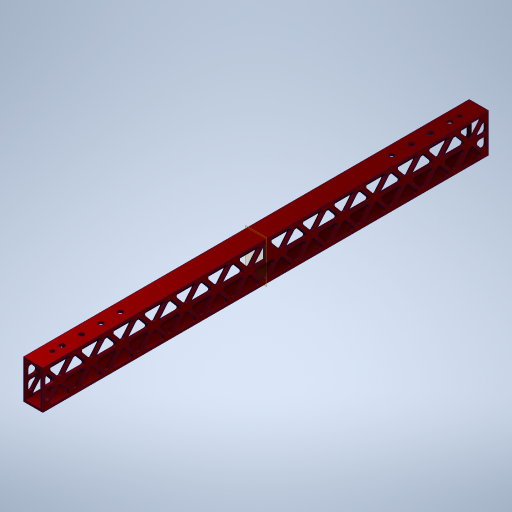
# Autodesk Inventor part: Drivetrain-Right-Left-Extrusion
Saved by Autodesk Inventor 2024.2 (Build 282272000, 272)
## iProperties
Created: 2024-01-04
Part Number: Drivetrain-Right-Left-Extrusion
Material: Aluminum 6061
Document SubType Name: Modeling
Designer: rohan
Density: 2.7 g/cm^3
Appearance: Aluminum - Flat
Author: rohan
Autodesk Inventor part; units mm, degrees
ref_plane "YZ Plane" through (0, 0, 0) normal (1, 0, 0) x (0, 1, 0)
ref_plane "XZ Plane" through (0, 0, 0) normal (0, 1, 0) x (-1, 0, 0)
ref_plane "XY Plane" through (0, 0, 0) normal (0, 0, 1) x (1, 0, 0)
sketch "Sketch1" plane through (0, 0, 0) normal (0, 0, 1) x (1, 0, 0)
  line L0 (-12.7, -25.4) -> (12.7, -25.4)
  line L1 (12.7, -25.4) -> (12.7, 25.4)
  line L2 (12.7, 25.4) -> (-12.7, 25.4)
  line L3 (-12.7, 25.4) -> (-12.7, -25.4)
  line L4 (-12.7, -25.4) -> (12.7, 25.4) construction
  line L5 (12.7, -25.4) -> (-12.7, 25.4) construction
  line L6 (-9.525, -22.225) -> (9.525, -22.225)
  line L7 (9.525, -22.225) -> (9.525, 22.225)
  line L8 (9.525, 22.225) -> (-9.525, 22.225)
  line L9 (-9.525, 22.225) -> (-9.525, -22.225)
  point P0 (0, 0)
  dimension "d0" = 25.4
  dimension "d1" = 50.8
  dimension "d2" = 3.175
  constraints: 20 end point, 4 parallel, 2 midpoint, 2 perpendicular, 1 horizontal, 3 other
  measures "d0" distance of L2.end L1.end
  measures "d1" distance of L1.end L0.end
  measures "d2" distance between parallel lines of L3 L9
extrude "Extrusion1" add sketch "Sketch1" along normal blind 584.2
sketch "Sketch2" plane through (-12.7, 25.4, 0) normal (0, 1, 0) x (1, 0, 0)
  circle A0 centre (12.7, -25.4) radius 2.5527
  circle A1 centre (12.7, -38.1) radius 3.2639
  line L0 (25.4, 0) -> (25.4, -584.2) projected
  circle A2 centre (12.7, -63.5) radius 3.2639
  circle A3 centre (12.7, -88.9) radius 3.2639
  circle A4 centre (12.7, -114.3) radius 3.2639
  point P0 (12.7, 0)
  dimension "d5" = 5.1054
  dimension "d6" = 25.4
  dimension "d7" = 6.5278
  dimension "d8" = 38.1
  dimension "d11" = 25.4
  constraints: 5 centre point, 1 vertical, 6 other
  measures "d5" diameter of A0
  measures "d6" distance of A0.centre point (12.7, 0)
  measures "d7" diameter of A1
  measures "d8" distance of A1.centre point (12.7, 0)
  measures "d11" distance of A1.centre A2.centre
extrude "Extrusion2" cut sketch "Sketch2" against normal blind 33.3375
ref_plane "Work Plane1" through (0, 0, 292.1) normal (0, 0, 1) x (1, 0, 0)
mirror "Mirror1" about plane through (0, 0, 292.1) normal (0, 0, 1) of "Extrusion2"
sketch "Sketch5" plane through (12.7, -25.4, 0) normal (1, 0, 0) x (0, 0, -1)
  line L0 (-584.2, 0) -> (-584.2, 50.8) projected
  line L1 (-584.2, 25.4) -> (0, 25.4)
  line L2 (-571.4463, 47.625) -> (-550.8435, 47.625)
  line L3 (-559.381, 30.6672) -> (-548.524, 42.2819)
  line L4 (0, 50.8) -> (-584.2, 50.8) projected
  line L5 (-564.1326, 30.7944) -> (-573.8785, 42.4091)
  arc A0 (-564.1326, 30.7944) -> (-559.381, 30.6672) centre (-561.7004, 32.8353) ccw
  arc A1 (-548.524, 42.2819) -> (-550.8435, 47.625) centre (-550.8435, 44.45) ccw
  arc A2 (-571.4463, 47.625) -> (-573.8785, 42.4091) centre (-571.4463, 44.45) ccw
  line L6 (-571.8917, 23.8125) -> (-577.85, 23.8125)
  line L7 (-569.4595, 18.5966) -> (-575.4178, 11.4958)
  line L8 (-581.025, 20.6375) -> (-581.025, 13.5367)
  line L9 (-571.8917, 26.9875) -> (-577.85, 26.9875)
  line L10 (-569.4595, 32.2034) -> (-575.4178, 39.3042)
  line L11 (-581.025, 30.1625) -> (-581.025, 37.2633)
  arc A3 (-575.4178, 39.3042) -> (-581.025, 37.2633) centre (-577.85, 37.2633) ccw
  arc A4 (-581.025, 30.1625) -> (-577.85, 26.9875) centre (-577.85, 30.1625) ccw
  arc A5 (-571.8917, 26.9875) -> (-569.4595, 32.2034) centre (-571.8917, 30.1625) ccw
  arc A6 (-577.85, 23.8125) -> (-581.025, 20.6375) centre (-577.85, 20.6375) ccw
  arc A7 (-569.4595, 18.5966) -> (-571.8917, 23.8125) centre (-571.8917, 20.6375) ccw
  arc A8 (-581.025, 13.5367) -> (-575.4178, 11.4958) centre (-577.85, 13.5367) ccw
  line L12 (-571.4463, 3.175) -> (-551.9485, 3.175)
  line L13 (-292.1, 50.8) -> (-292.1, 0)
  line L14 (0, 25.4) -> (-584.2, 25.4)
  line L15 (-542.6903, 6.0602) -> (-542.7392, 6.1185)
  line L16 (-564.1326, 20.0056) -> (-564.1356, 20.002)
  line L17 (-571.4463, 3.175) -> (-551.9605, 3.175)
  line L18 (-563.4572, 3.175) -> (-571.4463, 3.175)
  line L19 (-564.1356, 20.002) -> (-573.8785, 8.3909)
  line L20 (-559.2712, 20.002) -> (-549.5283, 8.3909)
  line L21 (-564.1356, 20.002) -> (-559.1614, 20.002) construction
  line L22 (-559.2712, 20.002) -> (-554.4261, 20.002) construction
  arc A9 (-573.8785, 8.3909) -> (-571.4463, 3.175) centre (-571.4463, 6.35) ccw
  arc A10 (-551.9605, 3.175) -> (-549.5283, 8.3909) centre (-551.9605, 6.35) ccw
  arc A11 (-559.2712, 20.002) -> (-564.1356, 20.002) centre (-561.7034, 17.9612) ccw
  line L23 (0, 0) -> (-584.2, 0) projected
  line L24 (-558.9257, 19.5902) -> (-549.5283, 8.3909)
  line L25 (-553.9473, 18.5966) -> (-547.0961, 10.4317)
  line L26 (-543.6299, 23.8125) -> (-551.5151, 23.8125)
  line L27 (-553.9473, 18.5966) -> (-544.208, 6.9898)
  line L28 (-543.6299, 23.8125) -> (-531.1495, 23.8125)
  line L29 (-551.5151, 23.8125) -> (-532.0365, 23.8125)
  line L30 (-529.6043, 18.5966) -> (-539.3436, 6.9898)
  arc A12 (-544.208, 6.9898) -> (-539.3436, 6.9898) centre (-541.7758, 9.0307) ccw
  arc A13 (-551.5151, 23.8125) -> (-553.9473, 18.5966) centre (-551.5151, 20.6375) ccw
  arc A14 (-529.6043, 18.5966) -> (-532.0365, 23.8125) centre (-532.0365, 20.6375) ccw
  line L31 (-557.5436, 23.8125) -> (-557.5862, 23.8125)
  line L32 (-558.2741, 23.8125) -> (-558.3239, 23.8125)
  line L33 (-553.9473, 32.2034) -> (-544.208, 43.8102)
  line L34 (-551.5151, 26.9875) -> (-532.0365, 26.9875)
  line L35 (-529.6043, 32.2034) -> (-539.3436, 43.8102)
  arc A15 (-539.3436, 43.8102) -> (-544.208, 43.8102) centre (-541.7758, 41.7693) ccw
  arc A16 (-553.9473, 32.2034) -> (-551.5151, 26.9875) centre (-551.5151, 30.1625) ccw
  arc A17 (-532.0365, 26.9875) -> (-529.6043, 32.2034) centre (-532.0365, 30.1625) ccw
  line L36 (-12.7537, 47.625) -> (-33.3565, 47.625)
  line L37 (-24.819, 30.6672) -> (-35.676, 42.2819)
  line L38 (-20.0674, 30.7944) -> (-10.3215, 42.4091)
  arc A18 (-24.819, 30.6672) -> (-20.0674, 30.7944) centre (-22.4996, 32.8353) ccw
  arc A19 (-33.3565, 47.625) -> (-35.676, 42.2819) centre (-33.3565, 44.45) ccw
  arc A20 (-10.3215, 42.4091) -> (-12.7537, 47.625) centre (-12.7537, 44.45) ccw
  line L39 (-12.3083, 23.8125) -> (-6.35, 23.8125)
  line L40 (-14.7405, 18.5966) -> (-8.7822, 11.4958)
  line L41 (-3.175, 20.6375) -> (-3.175, 13.5367)
  line L42 (-12.3083, 26.9875) -> (-6.35, 26.9875)
  line L43 (-3.175, 30.1625) -> (-3.175, 37.2633)
  line L44 (-14.7405, 32.2034) -> (-8.7822, 39.3042)
  arc A21 (-3.175, 37.2633) -> (-8.7822, 39.3042) centre (-6.35, 37.2633) ccw
  arc A22 (-6.35, 26.9875) -> (-3.175, 30.1625) centre (-6.35, 30.1625) ccw
  arc A23 (-14.7405, 32.2034) -> (-12.3083, 26.9875) centre (-12.3083, 30.1625) ccw
  arc A24 (-3.175, 20.6375) -> (-6.35, 23.8125) centre (-6.35, 20.6375) ccw
  arc A25 (-12.3083, 23.8125) -> (-14.7405, 18.5966) centre (-12.3083, 20.6375) ccw
  arc A26 (-8.7822, 11.4958) -> (-3.175, 13.5367) centre (-6.35, 13.5367) ccw
  line L45 (-12.7537, 3.175) -> (-32.2515, 3.175)
  line L46 (-20.0674, 20.0056) -> (-20.0644, 20.002)
  line L47 (-20.7428, 3.175) -> (-12.7537, 3.175)
  line L48 (-20.0644, 20.002) -> (-10.3215, 8.3909)
  line L49 (-24.9288, 20.002) -> (-34.6717, 8.3909)
  line L50 (-20.0644, 20.002) -> (-25.0386, 20.002) construction
  line L51 (-24.9288, 20.002) -> (-29.7739, 20.002) construction
  arc A27 (-12.7537, 3.175) -> (-10.3215, 8.3909) centre (-12.7537, 6.35) ccw
  arc A28 (-34.6717, 8.3909) -> (-32.2395, 3.175) centre (-32.2395, 6.35) ccw
  arc A29 (-20.0644, 20.002) -> (-24.9288, 20.002) centre (-22.4966, 17.9612) ccw
  line L52 (-26.6564, 23.8125) -> (-26.6138, 23.8125)
  line L53 (-25.9259, 23.8125) -> (-25.8761, 23.8125)
  line L54 (41.402, 25.4) -> (-542.798, 25.4)
  arc A30 (-522.7306, 30.7944) -> (-517.979, 30.6672) centre (-520.2984, 32.8353) ccw
  line L55 (-517.979, 30.6672) -> (-507.122, 42.2819)
  line L56 (-522.7306, 30.7944) -> (-532.4765, 42.4091)
  arc A31 (-507.122, 42.2819) -> (-509.4415, 47.625) centre (-509.4415, 44.45) ccw
  line L57 (-530.0443, 47.625) -> (-509.4415, 47.625)
  line L58 (-517.8692, 20.002) -> (-513.0241, 20.002) construction
  line L59 (-522.7336, 20.002) -> (-517.7594, 20.002) construction
  line L60 (-517.8692, 20.002) -> (-508.1263, 8.3909)
  arc A32 (-510.5585, 3.175) -> (-508.1263, 8.3909) centre (-510.5585, 6.35) ccw
  line L61 (-530.0443, 3.175) -> (-510.5465, 3.175)
  line L62 (-530.0443, 3.175) -> (-510.5585, 3.175)
  line L63 (-522.7336, 20.002) -> (-532.4765, 8.3909)
  line L64 (-522.0552, 3.175) -> (-530.0443, 3.175)
  arc A33 (-517.8692, 20.002) -> (-522.7336, 20.002) centre (-520.3014, 17.9612) ccw
  line L65 (-522.7306, 20.0056) -> (-522.7336, 20.002)
  line L66 (-501.2883, 6.0602) -> (-501.3372, 6.1185)
  line L67 (-517.5237, 19.5902) -> (-508.1263, 8.3909)
  line L68 (-512.5453, 18.5966) -> (-505.6941, 10.4317)
  line L69 (-502.2279, 23.8125) -> (-510.1131, 23.8125)
  line L70 (-512.5453, 18.5966) -> (-502.806, 6.9898)
  arc A34 (-488.2023, 18.5966) -> (-490.6345, 23.8125) centre (-490.6345, 20.6375) ccw
  arc A35 (-502.806, 6.9898) -> (-497.9416, 6.9898) centre (-500.3738, 9.0307) ccw
  line L71 (-488.2023, 18.5966) -> (-497.9416, 6.9898)
  line L72 (-502.2279, 23.8125) -> (-489.7475, 23.8125)
  arc A36 (-510.1131, 23.8125) -> (-512.5453, 18.5966) centre (-510.1131, 20.6375) ccw
  line L73 (-510.1131, 23.8125) -> (-490.6345, 23.8125)
  line L74 (-516.1416, 23.8125) -> (-516.1842, 23.8125)
  line L75 (-516.8721, 23.8125) -> (-516.9219, 23.8125)
  arc A37 (-490.6345, 26.9875) -> (-488.2023, 32.2034) centre (-490.6345, 30.1625) ccw
  line L76 (-510.1131, 26.9875) -> (-490.6345, 26.9875)
  arc A38 (-512.5453, 32.2034) -> (-510.1131, 26.9875) centre (-510.1131, 30.1625) ccw
  line L77 (-488.2023, 32.2034) -> (-497.9416, 43.8102)
  line L78 (-512.5453, 32.2034) -> (-502.806, 43.8102)
  arc A39 (-497.9416, 43.8102) -> (-502.806, 43.8102) centre (-500.3738, 41.7693) ccw
  arc A40 (-532.4765, 8.3909) -> (-530.0443, 3.175) centre (-530.0443, 6.35) ccw
  arc A41 (-530.0443, 47.625) -> (-532.4765, 42.4091) centre (-530.0443, 44.45) ccw
  line L79 (82.804, 25.4) -> (-501.396, 25.4)
  arc A42 (-481.3286, 30.7944) -> (-476.577, 30.6672) centre (-478.8964, 32.8353) ccw
  line L80 (-476.577, 30.6672) -> (-465.72, 42.2819)
  line L81 (-481.3286, 30.7944) -> (-491.0745, 42.4091)
  arc A43 (-465.72, 42.2819) -> (-468.0395, 47.625) centre (-468.0395, 44.45) ccw
  line L82 (-488.6423, 47.625) -> (-468.0395, 47.625)
  line L83 (-476.4672, 20.002) -> (-471.6221, 20.002) construction
  line L84 (-481.3316, 20.002) -> (-476.3574, 20.002) construction
  line L85 (-476.4672, 20.002) -> (-466.7243, 8.3909)
  arc A44 (-469.1565, 3.175) -> (-466.7243, 8.3909) centre (-469.1565, 6.35) ccw
  line L86 (-488.6423, 3.175) -> (-469.1445, 3.175)
  line L87 (-488.6423, 3.175) -> (-469.1565, 3.175)
  line L88 (-481.3316, 20.002) -> (-491.0745, 8.3909)
  line L89 (-480.6532, 3.175) -> (-488.6423, 3.175)
  arc A45 (-476.4672, 20.002) -> (-481.3316, 20.002) centre (-478.8994, 17.9612) ccw
  line L90 (-481.3286, 20.0056) -> (-481.3316, 20.002)
  line L91 (-459.8863, 6.0602) -> (-459.9352, 6.1185)
  line L92 (-476.1217, 19.5902) -> (-466.7243, 8.3909)
  line L93 (-471.1433, 18.5966) -> (-464.2921, 10.4317)
  line L94 (-460.8259, 23.8125) -> (-468.7111, 23.8125)
  line L95 (-471.1433, 18.5966) -> (-461.404, 6.9898)
  arc A46 (-446.8003, 18.5966) -> (-449.2325, 23.8125) centre (-449.2325, 20.6375) ccw
  arc A47 (-461.404, 6.9898) -> (-456.5396, 6.9898) centre (-458.9718, 9.0307) ccw
  line L96 (-446.8003, 18.5966) -> (-456.5396, 6.9898)
  line L97 (-460.8259, 23.8125) -> (-448.3455, 23.8125)
  arc A48 (-468.7111, 23.8125) -> (-471.1433, 18.5966) centre (-468.7111, 20.6375) ccw
  line L98 (-468.7111, 23.8125) -> (-449.2325, 23.8125)
  line L99 (-474.7396, 23.8125) -> (-474.7822, 23.8125)
  line L100 (-475.4701, 23.8125) -> (-475.5199, 23.8125)
  arc A49 (-449.2325, 26.9875) -> (-446.8003, 32.2034) centre (-449.2325, 30.1625) ccw
  line L101 (-468.7111, 26.9875) -> (-449.2325, 26.9875)
  arc A50 (-471.1433, 32.2034) -> (-468.7111, 26.9875) centre (-468.7111, 30.1625) ccw
  line L102 (-446.8003, 32.2034) -> (-456.5396, 43.8102)
  line L103 (-471.1433, 32.2034) -> (-461.404, 43.8102)
  arc A51 (-456.5396, 43.8102) -> (-461.404, 43.8102) centre (-458.9718, 41.7693) ccw
  arc A52 (-491.0745, 8.3909) -> (-488.6423, 3.175) centre (-488.6423, 6.35) ccw
  arc A53 (-488.6423, 47.625) -> (-491.0745, 42.4091) centre (-488.6423, 44.45) ccw
  line L104 (124.206, 25.4) -> (-459.994, 25.4)
  arc A54 (-439.9266, 30.7944) -> (-435.175, 30.6672) centre (-437.4944, 32.8353) ccw
  line L105 (-435.175, 30.6672) -> (-424.318, 42.2819)
  line L106 (-439.9266, 30.7944) -> (-449.6725, 42.4091)
  arc A55 (-424.318, 42.2819) -> (-426.6375, 47.625) centre (-426.6375, 44.45) ccw
  line L107 (-447.2403, 47.625) -> (-426.6375, 47.625)
  line L108 (-435.0652, 20.002) -> (-430.2201, 20.002) construction
  line L109 (-439.9296, 20.002) -> (-434.9554, 20.002) construction
  line L110 (-435.0652, 20.002) -> (-425.3223, 8.3909)
  arc A56 (-427.7545, 3.175) -> (-425.3223, 8.3909) centre (-427.7545, 6.35) ccw
  line L111 (-447.2403, 3.175) -> (-427.7425, 3.175)
  line L112 (-447.2403, 3.175) -> (-427.7545, 3.175)
  line L113 (-439.9296, 20.002) -> (-449.6725, 8.3909)
  line L114 (-439.2512, 3.175) -> (-447.2403, 3.175)
  arc A57 (-435.0652, 20.002) -> (-439.9296, 20.002) centre (-437.4974, 17.9612) ccw
  line L115 (-439.9266, 20.0056) -> (-439.9296, 20.002)
  line L116 (-418.4843, 6.0602) -> (-418.5332, 6.1185)
  line L117 (-434.7197, 19.5902) -> (-425.3223, 8.3909)
  line L118 (-429.7413, 18.5966) -> (-422.8901, 10.4317)
  line L119 (-419.4239, 23.8125) -> (-427.3091, 23.8125)
  line L120 (-429.7413, 18.5966) -> (-420.002, 6.9898)
  arc A58 (-405.3983, 18.5966) -> (-407.8305, 23.8125) centre (-407.8305, 20.6375) ccw
  arc A59 (-420.002, 6.9898) -> (-415.1376, 6.9898) centre (-417.5698, 9.0307) ccw
  line L121 (-405.3983, 18.5966) -> (-415.1376, 6.9898)
  line L122 (-419.4239, 23.8125) -> (-406.9435, 23.8125)
  arc A60 (-427.3091, 23.8125) -> (-429.7413, 18.5966) centre (-427.3091, 20.6375) ccw
  line L123 (-427.3091, 23.8125) -> (-407.8305, 23.8125)
  line L124 (-433.3376, 23.8125) -> (-433.3802, 23.8125)
  line L125 (-434.0681, 23.8125) -> (-434.1179, 23.8125)
  arc A61 (-407.8305, 26.9875) -> (-405.3983, 32.2034) centre (-407.8305, 30.1625) ccw
  line L126 (-427.3091, 26.9875) -> (-407.8305, 26.9875)
  arc A62 (-429.7413, 32.2034) -> (-427.3091, 26.9875) centre (-427.3091, 30.1625) ccw
  line L127 (-405.3983, 32.2034) -> (-415.1376, 43.8102)
  line L128 (-429.7413, 32.2034) -> (-420.002, 43.8102)
  arc A63 (-415.1376, 43.8102) -> (-420.002, 43.8102) centre (-417.5698, 41.7693) ccw
  arc A64 (-449.6725, 8.3909) -> (-447.2403, 3.175) centre (-447.2403, 6.35) ccw
  arc A65 (-447.2403, 47.625) -> (-449.6725, 42.4091) centre (-447.2403, 44.45) ccw
  line L129 (165.608, 25.4) -> (-418.592, 25.4)
  arc A66 (-398.5246, 30.7944) -> (-393.773, 30.6672) centre (-396.0924, 32.8353) ccw
  line L130 (-393.773, 30.6672) -> (-382.916, 42.2819)
  line L131 (-398.5246, 30.7944) -> (-408.2705, 42.4091)
  arc A67 (-382.916, 42.2819) -> (-385.2355, 47.625) centre (-385.2355, 44.45) ccw
  line L132 (-405.8383, 47.625) -> (-385.2355, 47.625)
  line L133 (-393.6632, 20.002) -> (-388.8181, 20.002) construction
  line L134 (-398.5276, 20.002) -> (-393.5534, 20.002) construction
  line L135 (-393.6632, 20.002) -> (-383.9203, 8.3909)
  arc A68 (-386.3525, 3.175) -> (-383.9203, 8.3909) centre (-386.3525, 6.35) ccw
  line L136 (-405.8383, 3.175) -> (-386.3405, 3.175)
  line L137 (-405.8383, 3.175) -> (-386.3525, 3.175)
  line L138 (-398.5276, 20.002) -> (-408.2705, 8.3909)
  line L139 (-397.8492, 3.175) -> (-405.8383, 3.175)
  arc A69 (-393.6632, 20.002) -> (-398.5276, 20.002) centre (-396.0954, 17.9612) ccw
  line L140 (-398.5246, 20.0056) -> (-398.5276, 20.002)
  line L141 (-377.0823, 6.0602) -> (-377.1312, 6.1185)
  line L142 (-393.3177, 19.5902) -> (-383.9203, 8.3909)
  line L143 (-388.3393, 18.5966) -> (-381.4881, 10.4317)
  line L144 (-378.0219, 23.8125) -> (-385.9071, 23.8125)
  line L145 (-388.3393, 18.5966) -> (-378.6, 6.9898)
  arc A70 (-363.9963, 18.5966) -> (-366.4285, 23.8125) centre (-366.4285, 20.6375) ccw
  arc A71 (-378.6, 6.9898) -> (-373.7356, 6.9898) centre (-376.1678, 9.0307) ccw
  line L146 (-363.9963, 18.5966) -> (-373.7356, 6.9898)
  line L147 (-378.0219, 23.8125) -> (-365.5415, 23.8125)
  arc A72 (-385.9071, 23.8125) -> (-388.3393, 18.5966) centre (-385.9071, 20.6375) ccw
  line L148 (-385.9071, 23.8125) -> (-366.4285, 23.8125)
  line L149 (-391.9356, 23.8125) -> (-391.9782, 23.8125)
  line L150 (-392.6661, 23.8125) -> (-392.7159, 23.8125)
  arc A73 (-366.4285, 26.9875) -> (-363.9963, 32.2034) centre (-366.4285, 30.1625) ccw
  line L151 (-385.9071, 26.9875) -> (-366.4285, 26.9875)
  arc A74 (-388.3393, 32.2034) -> (-385.9071, 26.9875) centre (-385.9071, 30.1625) ccw
  line L152 (-363.9963, 32.2034) -> (-373.7356, 43.8102)
  line L153 (-388.3393, 32.2034) -> (-378.6, 43.8102)
  arc A75 (-373.7356, 43.8102) -> (-378.6, 43.8102) centre (-376.1678, 41.7693) ccw
  arc A76 (-408.2705, 8.3909) -> (-405.8383, 3.175) centre (-405.8383, 6.35) ccw
  arc A77 (-405.8383, 47.625) -> (-408.2705, 42.4091) centre (-405.8383, 44.45) ccw
  line L154 (207.01, 25.4) -> (-377.19, 25.4)
  arc A78 (-357.1226, 30.7944) -> (-352.371, 30.6672) centre (-354.6904, 32.8353) ccw
  line L155 (-352.371, 30.6672) -> (-341.514, 42.2819)
  line L156 (-357.1226, 30.7944) -> (-366.8685, 42.4091)
  arc A79 (-341.514, 42.2819) -> (-343.8335, 47.625) centre (-343.8335, 44.45) ccw
  line L157 (-364.4363, 47.625) -> (-343.8335, 47.625)
  line L158 (-352.2612, 20.002) -> (-347.4161, 20.002) construction
  line L159 (-357.1256, 20.002) -> (-352.1514, 20.002) construction
  line L160 (-352.2612, 20.002) -> (-342.5183, 8.3909)
  arc A80 (-344.9505, 3.175) -> (-342.5183, 8.3909) centre (-344.9505, 6.35) ccw
  line L161 (-364.4363, 3.175) -> (-344.9385, 3.175)
  line L162 (-364.4363, 3.175) -> (-344.9505, 3.175)
  line L163 (-357.1256, 20.002) -> (-366.8685, 8.3909)
  line L164 (-356.4472, 3.175) -> (-364.4363, 3.175)
  arc A81 (-352.2612, 20.002) -> (-357.1256, 20.002) centre (-354.6934, 17.9612) ccw
  line L165 (-357.1226, 20.0056) -> (-357.1256, 20.002)
  line L166 (-335.6803, 6.0602) -> (-335.7292, 6.1185)
  line L167 (-351.9157, 19.5902) -> (-342.5183, 8.3909)
  line L168 (-346.9373, 18.5966) -> (-340.0861, 10.4317)
  line L169 (-336.6199, 23.8125) -> (-344.5051, 23.8125)
  line L170 (-346.9373, 18.5966) -> (-337.198, 6.9898)
  arc A82 (-322.5943, 18.5966) -> (-325.0265, 23.8125) centre (-325.0265, 20.6375) ccw
  arc A83 (-337.198, 6.9898) -> (-332.3336, 6.9898) centre (-334.7658, 9.0307) ccw
  line L171 (-322.5943, 18.5966) -> (-332.3336, 6.9898)
  line L172 (-336.6199, 23.8125) -> (-324.1395, 23.8125)
  arc A84 (-344.5051, 23.8125) -> (-346.9373, 18.5966) centre (-344.5051, 20.6375) ccw
  line L173 (-344.5051, 23.8125) -> (-325.0265, 23.8125)
  line L174 (-350.5336, 23.8125) -> (-350.5762, 23.8125)
  line L175 (-351.2641, 23.8125) -> (-351.3139, 23.8125)
  arc A85 (-325.0265, 26.9875) -> (-322.5943, 32.2034) centre (-325.0265, 30.1625) ccw
  line L176 (-344.5051, 26.9875) -> (-325.0265, 26.9875)
  arc A86 (-346.9373, 32.2034) -> (-344.5051, 26.9875) centre (-344.5051, 30.1625) ccw
  line L177 (-322.5943, 32.2034) -> (-332.3336, 43.8102)
  line L178 (-346.9373, 32.2034) -> (-337.198, 43.8102)
  arc A87 (-332.3336, 43.8102) -> (-337.198, 43.8102) centre (-334.7658, 41.7693) ccw
  arc A88 (-366.8685, 8.3909) -> (-364.4363, 3.175) centre (-364.4363, 6.35) ccw
  arc A89 (-364.4363, 47.625) -> (-366.8685, 42.4091) centre (-364.4363, 44.45) ccw
  line L179 (248.412, 25.4) -> (-335.788, 25.4)
  arc A90 (-315.7206, 30.7944) -> (-310.969, 30.6672) centre (-313.2884, 32.8353) ccw
  line L180 (-310.969, 30.6672) -> (-300.112, 42.2819)
  line L181 (-315.7206, 30.7944) -> (-325.4665, 42.4091)
  arc A91 (-300.112, 42.2819) -> (-302.4315, 47.625) centre (-302.4315, 44.45) ccw
  line L182 (-323.0343, 47.625) -> (-302.4315, 47.625)
  line L183 (-310.8592, 20.002) -> (-306.0141, 20.002) construction
  line L184 (-315.7236, 20.002) -> (-310.7494, 20.002) construction
  line L185 (-310.8592, 20.002) -> (-301.1163, 8.3909)
  arc A92 (-303.5485, 3.175) -> (-301.1163, 8.3909) centre (-303.5485, 6.35) ccw
  line L186 (-323.0343, 3.175) -> (-303.5365, 3.175)
  line L187 (-323.0343, 3.175) -> (-303.5485, 3.175)
  line L188 (-315.7236, 20.002) -> (-325.4665, 8.3909)
  line L189 (-315.0452, 3.175) -> (-323.0343, 3.175)
  arc A93 (-310.8592, 20.002) -> (-315.7236, 20.002) centre (-313.2914, 17.9612) ccw
  line L190 (-315.7206, 20.0056) -> (-315.7236, 20.002)
  line L191 (-294.2783, 6.0602) -> (-294.3272, 6.1185)
  line L192 (-310.5137, 19.5902) -> (-301.1163, 8.3909)
  line L193 (-305.5353, 18.5966) -> (-298.6841, 10.4317)
  line L194 (-295.2179, 23.8125) -> (-303.1031, 23.8125)
  line L195 (-305.5353, 18.5966) -> (-295.796, 6.9898)
  arc A94 (-281.1923, 18.5966) -> (-283.6245, 23.8125) centre (-283.6245, 20.6375) ccw
  arc A95 (-295.796, 6.9898) -> (-290.9316, 6.9898) centre (-293.3638, 9.0307) ccw
  line L196 (-281.1923, 18.5966) -> (-290.9316, 6.9898)
  line L197 (-295.2179, 23.8125) -> (-282.7375, 23.8125)
  arc A96 (-303.1031, 23.8125) -> (-305.5353, 18.5966) centre (-303.1031, 20.6375) ccw
  line L198 (-303.1031, 23.8125) -> (-283.6245, 23.8125)
  line L199 (-309.1316, 23.8125) -> (-309.1742, 23.8125)
  line L200 (-309.8621, 23.8125) -> (-309.9119, 23.8125)
  arc A97 (-283.6245, 26.9875) -> (-281.1923, 32.2034) centre (-283.6245, 30.1625) ccw
  line L201 (-303.1031, 26.9875) -> (-283.6245, 26.9875)
  arc A98 (-305.5353, 32.2034) -> (-303.1031, 26.9875) centre (-303.1031, 30.1625) ccw
  line L202 (-281.1923, 32.2034) -> (-290.9316, 43.8102)
  line L203 (-305.5353, 32.2034) -> (-295.796, 43.8102)
  arc A99 (-290.9316, 43.8102) -> (-295.796, 43.8102) centre (-293.3638, 41.7693) ccw
  arc A100 (-325.4665, 8.3909) -> (-323.0343, 3.175) centre (-323.0343, 6.35) ccw
  arc A101 (-323.0343, 47.625) -> (-325.4665, 42.4091) centre (-323.0343, 44.45) ccw
  line L204 (289.814, 25.4) -> (-294.386, 25.4)
  arc A102 (-274.3186, 30.7944) -> (-269.567, 30.6672) centre (-271.8864, 32.8353) ccw
  line L205 (-269.567, 30.6672) -> (-258.71, 42.2819)
  line L206 (-274.3186, 30.7944) -> (-284.0645, 42.4091)
  arc A103 (-258.71, 42.2819) -> (-261.0295, 47.625) centre (-261.0295, 44.45) ccw
  line L207 (-281.6323, 47.625) -> (-261.0295, 47.625)
  line L208 (-269.4572, 20.002) -> (-264.6121, 20.002) construction
  line L209 (-274.3216, 20.002) -> (-269.3474, 20.002) construction
  line L210 (-269.4572, 20.002) -> (-259.7143, 8.3909)
  arc A104 (-262.1465, 3.175) -> (-259.7143, 8.3909) centre (-262.1465, 6.35) ccw
  line L211 (-281.6323, 3.175) -> (-262.1345, 3.175)
  line L212 (-281.6323, 3.175) -> (-262.1465, 3.175)
  line L213 (-274.3216, 20.002) -> (-284.0645, 8.3909)
  line L214 (-273.6432, 3.175) -> (-281.6323, 3.175)
  arc A105 (-269.4572, 20.002) -> (-274.3216, 20.002) centre (-271.8894, 17.9612) ccw
  line L215 (-274.3186, 20.0056) -> (-274.3216, 20.002)
  line L216 (-252.8763, 6.0602) -> (-252.9252, 6.1185)
  line L217 (-269.1117, 19.5902) -> (-259.7143, 8.3909)
  line L218 (-264.1333, 18.5966) -> (-257.2821, 10.4317)
  line L219 (-253.8159, 23.8125) -> (-261.7011, 23.8125)
  line L220 (-264.1333, 18.5966) -> (-254.394, 6.9898)
  arc A106 (-239.7903, 18.5966) -> (-242.2225, 23.8125) centre (-242.2225, 20.6375) ccw
  arc A107 (-254.394, 6.9898) -> (-249.5296, 6.9898) centre (-251.9618, 9.0307) ccw
  line L221 (-239.7903, 18.5966) -> (-249.5296, 6.9898)
  line L222 (-253.8159, 23.8125) -> (-241.3355, 23.8125)
  arc A108 (-261.7011, 23.8125) -> (-264.1333, 18.5966) centre (-261.7011, 20.6375) ccw
  line L223 (-261.7011, 23.8125) -> (-242.2225, 23.8125)
  line L224 (-267.7296, 23.8125) -> (-267.7722, 23.8125)
  line L225 (-268.4601, 23.8125) -> (-268.5099, 23.8125)
  arc A109 (-242.2225, 26.9875) -> (-239.7903, 32.2034) centre (-242.2225, 30.1625) ccw
  line L226 (-261.7011, 26.9875) -> (-242.2225, 26.9875)
  arc A110 (-264.1333, 32.2034) -> (-261.7011, 26.9875) centre (-261.7011, 30.1625) ccw
  line L227 (-239.7903, 32.2034) -> (-249.5296, 43.8102)
  line L228 (-264.1333, 32.2034) -> (-254.394, 43.8102)
  arc A111 (-249.5296, 43.8102) -> (-254.394, 43.8102) centre (-251.9618, 41.7693) ccw
  arc A112 (-284.0645, 8.3909) -> (-281.6323, 3.175) centre (-281.6323, 6.35) ccw
  arc A113 (-281.6323, 47.625) -> (-284.0645, 42.4091) centre (-281.6323, 44.45) ccw
  line L229 (331.216, 25.4) -> (-252.984, 25.4)
  arc A114 (-232.9166, 30.7944) -> (-228.165, 30.6672) centre (-230.4844, 32.8353) ccw
  line L230 (-228.165, 30.6672) -> (-217.308, 42.2819)
  line L231 (-232.9166, 30.7944) -> (-242.6625, 42.4091)
  arc A115 (-217.308, 42.2819) -> (-219.6275, 47.625) centre (-219.6275, 44.45) ccw
  line L232 (-240.2303, 47.625) -> (-219.6275, 47.625)
  line L233 (-228.0552, 20.002) -> (-223.2101, 20.002) construction
  line L234 (-232.9196, 20.002) -> (-227.9454, 20.002) construction
  line L235 (-228.0552, 20.002) -> (-218.3123, 8.3909)
  arc A116 (-220.7445, 3.175) -> (-218.3123, 8.3909) centre (-220.7445, 6.35) ccw
  line L236 (-240.2303, 3.175) -> (-220.7325, 3.175)
  line L237 (-240.2303, 3.175) -> (-220.7445, 3.175)
  line L238 (-232.9196, 20.002) -> (-242.6625, 8.3909)
  line L239 (-232.2412, 3.175) -> (-240.2303, 3.175)
  arc A117 (-228.0552, 20.002) -> (-232.9196, 20.002) centre (-230.4874, 17.9612) ccw
  line L240 (-232.9166, 20.0056) -> (-232.9196, 20.002)
  line L241 (-211.4743, 6.0602) -> (-211.5232, 6.1185)
  line L242 (-227.7097, 19.5902) -> (-218.3123, 8.3909)
  line L243 (-222.7313, 18.5966) -> (-215.8801, 10.4317)
  line L244 (-212.4139, 23.8125) -> (-220.2991, 23.8125)
  line L245 (-222.7313, 18.5966) -> (-212.992, 6.9898)
  arc A118 (-198.3883, 18.5966) -> (-200.8205, 23.8125) centre (-200.8205, 20.6375) ccw
  arc A119 (-212.992, 6.9898) -> (-208.1276, 6.9898) centre (-210.5598, 9.0307) ccw
  line L246 (-198.3883, 18.5966) -> (-208.1276, 6.9898)
  line L247 (-212.4139, 23.8125) -> (-199.9335, 23.8125)
  arc A120 (-220.2991, 23.8125) -> (-222.7313, 18.5966) centre (-220.2991, 20.6375) ccw
  line L248 (-220.2991, 23.8125) -> (-200.8205, 23.8125)
  line L249 (-226.3276, 23.8125) -> (-226.3702, 23.8125)
  line L250 (-227.0581, 23.8125) -> (-227.1079, 23.8125)
  arc A121 (-200.8205, 26.9875) -> (-198.3883, 32.2034) centre (-200.8205, 30.1625) ccw
  line L251 (-220.2991, 26.9875) -> (-200.8205, 26.9875)
  arc A122 (-222.7313, 32.2034) -> (-220.2991, 26.9875) centre (-220.2991, 30.1625) ccw
  line L252 (-198.3883, 32.2034) -> (-208.1276, 43.8102)
  line L253 (-222.7313, 32.2034) -> (-212.992, 43.8102)
  arc A123 (-208.1276, 43.8102) -> (-212.992, 43.8102) centre (-210.5598, 41.7693) ccw
  arc A124 (-242.6625, 8.3909) -> (-240.2303, 3.175) centre (-240.2303, 6.35) ccw
  arc A125 (-240.2303, 47.625) -> (-242.6625, 42.4091) centre (-240.2303, 44.45) ccw
  line L254 (372.618, 25.4) -> (-211.582, 25.4)
  arc A126 (-191.5146, 30.7944) -> (-186.763, 30.6672) centre (-189.0824, 32.8353) ccw
  line L255 (-186.763, 30.6672) -> (-175.906, 42.2819)
  line L256 (-191.5146, 30.7944) -> (-201.2605, 42.4091)
  arc A127 (-175.906, 42.2819) -> (-178.2255, 47.625) centre (-178.2255, 44.45) ccw
  line L257 (-198.8283, 47.625) -> (-178.2255, 47.625)
  line L258 (-186.6532, 20.002) -> (-181.8081, 20.002) construction
  line L259 (-191.5176, 20.002) -> (-186.5434, 20.002) construction
  line L260 (-186.6532, 20.002) -> (-176.9103, 8.3909)
  arc A128 (-179.3425, 3.175) -> (-176.9103, 8.3909) centre (-179.3425, 6.35) ccw
  line L261 (-198.8283, 3.175) -> (-179.3305, 3.175)
  line L262 (-198.8283, 3.175) -> (-179.3425, 3.175)
  line L263 (-191.5176, 20.002) -> (-201.2605, 8.3909)
  line L264 (-190.8392, 3.175) -> (-198.8283, 3.175)
  arc A129 (-186.6532, 20.002) -> (-191.5176, 20.002) centre (-189.0854, 17.9612) ccw
  line L265 (-191.5146, 20.0056) -> (-191.5176, 20.002)
  line L266 (-170.0723, 6.0602) -> (-170.1212, 6.1185)
  line L267 (-186.3077, 19.5902) -> (-176.9103, 8.3909)
  line L268 (-181.3293, 18.5966) -> (-174.4781, 10.4317)
  line L269 (-171.0119, 23.8125) -> (-178.8971, 23.8125)
  line L270 (-181.3293, 18.5966) -> (-171.59, 6.9898)
  arc A130 (-156.9863, 18.5966) -> (-159.4185, 23.8125) centre (-159.4185, 20.6375) ccw
  arc A131 (-171.59, 6.9898) -> (-166.7256, 6.9898) centre (-169.1578, 9.0307) ccw
  line L271 (-156.9863, 18.5966) -> (-166.7256, 6.9898)
  line L272 (-171.0119, 23.8125) -> (-158.5315, 23.8125)
  arc A132 (-178.8971, 23.8125) -> (-181.3293, 18.5966) centre (-178.8971, 20.6375) ccw
  line L273 (-178.8971, 23.8125) -> (-159.4185, 23.8125)
  line L274 (-184.9256, 23.8125) -> (-184.9682, 23.8125)
  line L275 (-185.6561, 23.8125) -> (-185.7059, 23.8125)
  arc A133 (-159.4185, 26.9875) -> (-156.9863, 32.2034) centre (-159.4185, 30.1625) ccw
  line L276 (-178.8971, 26.9875) -> (-159.4185, 26.9875)
  arc A134 (-181.3293, 32.2034) -> (-178.8971, 26.9875) centre (-178.8971, 30.1625) ccw
  line L277 (-156.9863, 32.2034) -> (-166.7256, 43.8102)
  line L278 (-181.3293, 32.2034) -> (-171.59, 43.8102)
  arc A135 (-166.7256, 43.8102) -> (-171.59, 43.8102) centre (-169.1578, 41.7693) ccw
  arc A136 (-201.2605, 8.3909) -> (-198.8283, 3.175) centre (-198.8283, 6.35) ccw
  arc A137 (-198.8283, 47.625) -> (-201.2605, 42.4091) centre (-198.8283, 44.45) ccw
  line L279 (414.02, 25.4) -> (-170.18, 25.4)
  arc A138 (-150.1126, 30.7944) -> (-145.361, 30.6672) centre (-147.6804, 32.8353) ccw
  line L280 (-145.361, 30.6672) -> (-134.504, 42.2819)
  line L281 (-150.1126, 30.7944) -> (-159.8585, 42.4091)
  arc A139 (-134.504, 42.2819) -> (-136.8235, 47.625) centre (-136.8235, 44.45) ccw
  line L282 (-157.4263, 47.625) -> (-136.8235, 47.625)
  line L283 (-145.2512, 20.002) -> (-140.4061, 20.002) construction
  line L284 (-150.1156, 20.002) -> (-145.1414, 20.002) construction
  line L285 (-145.2512, 20.002) -> (-135.5083, 8.3909)
  arc A140 (-137.9405, 3.175) -> (-135.5083, 8.3909) centre (-137.9405, 6.35) ccw
  line L286 (-157.4263, 3.175) -> (-137.9285, 3.175)
  line L287 (-157.4263, 3.175) -> (-137.9405, 3.175)
  line L288 (-150.1156, 20.002) -> (-159.8585, 8.3909)
  line L289 (-149.4372, 3.175) -> (-157.4263, 3.175)
  arc A141 (-145.2512, 20.002) -> (-150.1156, 20.002) centre (-147.6834, 17.9612) ccw
  line L290 (-150.1126, 20.0056) -> (-150.1156, 20.002)
  line L291 (-128.6703, 6.0602) -> (-128.7192, 6.1185)
  line L292 (-144.9057, 19.5902) -> (-135.5083, 8.3909)
  line L293 (-139.9273, 18.5966) -> (-133.0761, 10.4317)
  line L294 (-129.6099, 23.8125) -> (-137.4951, 23.8125)
  line L295 (-139.9273, 18.5966) -> (-130.188, 6.9898)
  arc A142 (-115.5843, 18.5966) -> (-118.0165, 23.8125) centre (-118.0165, 20.6375) ccw
  arc A143 (-130.188, 6.9898) -> (-125.3236, 6.9898) centre (-127.7558, 9.0307) ccw
  line L296 (-115.5843, 18.5966) -> (-125.3236, 6.9898)
  line L297 (-129.6099, 23.8125) -> (-117.1295, 23.8125)
  arc A144 (-137.4951, 23.8125) -> (-139.9273, 18.5966) centre (-137.4951, 20.6375) ccw
  line L298 (-137.4951, 23.8125) -> (-118.0165, 23.8125)
  line L299 (-143.5236, 23.8125) -> (-143.5662, 23.8125)
  line L300 (-144.2541, 23.8125) -> (-144.3039, 23.8125)
  arc A145 (-118.0165, 26.9875) -> (-115.5843, 32.2034) centre (-118.0165, 30.1625) ccw
  line L301 (-137.4951, 26.9875) -> (-118.0165, 26.9875)
  arc A146 (-139.9273, 32.2034) -> (-137.4951, 26.9875) centre (-137.4951, 30.1625) ccw
  line L302 (-115.5843, 32.2034) -> (-125.3236, 43.8102)
  line L303 (-139.9273, 32.2034) -> (-130.188, 43.8102)
  arc A147 (-125.3236, 43.8102) -> (-130.188, 43.8102) centre (-127.7558, 41.7693) ccw
  arc A148 (-159.8585, 8.3909) -> (-157.4263, 3.175) centre (-157.4263, 6.35) ccw
  arc A149 (-157.4263, 47.625) -> (-159.8585, 42.4091) centre (-157.4263, 44.45) ccw
  line L304 (455.422, 25.4) -> (-128.778, 25.4)
  arc A150 (-108.7106, 30.7944) -> (-103.959, 30.6672) centre (-106.2784, 32.8353) ccw
  line L305 (-103.959, 30.6672) -> (-93.102, 42.2819)
  line L306 (-108.7106, 30.7944) -> (-118.4565, 42.4091)
  arc A151 (-93.102, 42.2819) -> (-95.4215, 47.625) centre (-95.4215, 44.45) ccw
  line L307 (-116.0243, 47.625) -> (-95.4215, 47.625)
  line L308 (-103.8492, 20.002) -> (-99.0041, 20.002) construction
  line L309 (-108.7136, 20.002) -> (-103.7394, 20.002) construction
  line L310 (-103.8492, 20.002) -> (-94.1063, 8.3909)
  arc A152 (-96.5385, 3.175) -> (-94.1063, 8.3909) centre (-96.5385, 6.35) ccw
  line L311 (-116.0243, 3.175) -> (-96.5265, 3.175)
  line L312 (-116.0243, 3.175) -> (-96.5385, 3.175)
  line L313 (-108.7136, 20.002) -> (-118.4565, 8.3909)
  line L314 (-108.0352, 3.175) -> (-116.0243, 3.175)
  arc A153 (-103.8492, 20.002) -> (-108.7136, 20.002) centre (-106.2814, 17.9612) ccw
  line L315 (-108.7106, 20.0056) -> (-108.7136, 20.002)
  line L316 (-87.2683, 6.0602) -> (-87.3172, 6.1185)
  line L317 (-103.5037, 19.5902) -> (-94.1063, 8.3909)
  line L318 (-98.5253, 18.5966) -> (-91.6741, 10.4317)
  line L319 (-88.2079, 23.8125) -> (-96.0931, 23.8125)
  line L320 (-98.5253, 18.5966) -> (-88.786, 6.9898)
  arc A154 (-74.1823, 18.5966) -> (-76.6145, 23.8125) centre (-76.6145, 20.6375) ccw
  arc A155 (-88.786, 6.9898) -> (-83.9216, 6.9898) centre (-86.3538, 9.0307) ccw
  line L321 (-74.1823, 18.5966) -> (-83.9216, 6.9898)
  line L322 (-88.2079, 23.8125) -> (-75.7275, 23.8125)
  arc A156 (-96.0931, 23.8125) -> (-98.5253, 18.5966) centre (-96.0931, 20.6375) ccw
  line L323 (-96.0931, 23.8125) -> (-76.6145, 23.8125)
  line L324 (-102.1216, 23.8125) -> (-102.1642, 23.8125)
  line L325 (-102.8521, 23.8125) -> (-102.9019, 23.8125)
  arc A157 (-76.6145, 26.9875) -> (-74.1823, 32.2034) centre (-76.6145, 30.1625) ccw
  line L326 (-96.0931, 26.9875) -> (-76.6145, 26.9875)
  arc A158 (-98.5253, 32.2034) -> (-96.0931, 26.9875) centre (-96.0931, 30.1625) ccw
  line L327 (-74.1823, 32.2034) -> (-83.9216, 43.8102)
  line L328 (-98.5253, 32.2034) -> (-88.786, 43.8102)
  arc A159 (-83.9216, 43.8102) -> (-88.786, 43.8102) centre (-86.3538, 41.7693) ccw
  arc A160 (-118.4565, 8.3909) -> (-116.0243, 3.175) centre (-116.0243, 6.35) ccw
  arc A161 (-116.0243, 47.625) -> (-118.4565, 42.4091) centre (-116.0243, 44.45) ccw
  line L329 (496.824, 25.4) -> (-87.376, 25.4)
  arc A162 (-67.3086, 30.7944) -> (-62.557, 30.6672) centre (-64.8764, 32.8353) ccw
  line L330 (-62.557, 30.6672) -> (-51.7, 42.2819)
  line L331 (-67.3086, 30.7944) -> (-77.0545, 42.4091)
  arc A163 (-51.7, 42.2819) -> (-54.0195, 47.625) centre (-54.0195, 44.45) ccw
  line L332 (-74.6223, 47.625) -> (-54.0195, 47.625)
  line L333 (-62.4472, 20.002) -> (-57.6021, 20.002) construction
  line L334 (-67.3116, 20.002) -> (-62.3374, 20.002) construction
  line L335 (-62.4472, 20.002) -> (-52.7043, 8.3909)
  arc A164 (-55.1365, 3.175) -> (-52.7043, 8.3909) centre (-55.1365, 6.35) ccw
  line L336 (-74.6223, 3.175) -> (-55.1245, 3.175)
  line L337 (-74.6223, 3.175) -> (-55.1365, 3.175)
  line L338 (-67.3116, 20.002) -> (-77.0545, 8.3909)
  line L339 (-66.6332, 3.175) -> (-74.6223, 3.175)
  arc A165 (-62.4472, 20.002) -> (-67.3116, 20.002) centre (-64.8794, 17.9612) ccw
  line L340 (-67.3086, 20.0056) -> (-67.3116, 20.002)
  line L341 (-45.8663, 6.0602) -> (-45.9152, 6.1185)
  line L342 (-62.1017, 19.5902) -> (-52.7043, 8.3909)
  line L343 (-57.1233, 18.5966) -> (-50.2721, 10.4317)
  line L344 (-46.8059, 23.8125) -> (-54.6911, 23.8125)
  line L345 (-57.1233, 18.5966) -> (-47.384, 6.9898)
  arc A166 (-32.7803, 18.5966) -> (-35.2125, 23.8125) centre (-35.2125, 20.6375) ccw
  arc A167 (-47.384, 6.9898) -> (-42.5196, 6.9898) centre (-44.9518, 9.0307) ccw
  line L346 (-32.7803, 18.5966) -> (-42.5196, 6.9898)
  line L347 (-46.8059, 23.8125) -> (-34.3255, 23.8125)
  arc A168 (-54.6911, 23.8125) -> (-57.1233, 18.5966) centre (-54.6911, 20.6375) ccw
  line L348 (-54.6911, 23.8125) -> (-35.2125, 23.8125)
  line L349 (-60.7196, 23.8125) -> (-60.7622, 23.8125)
  line L350 (-61.4501, 23.8125) -> (-61.4999, 23.8125)
  arc A169 (-35.2125, 26.9875) -> (-32.7803, 32.2034) centre (-35.2125, 30.1625) ccw
  line L351 (-54.6911, 26.9875) -> (-35.2125, 26.9875)
  arc A170 (-57.1233, 32.2034) -> (-54.6911, 26.9875) centre (-54.6911, 30.1625) ccw
  line L352 (-32.7803, 32.2034) -> (-42.5196, 43.8102)
  line L353 (-57.1233, 32.2034) -> (-47.384, 43.8102)
  arc A171 (-42.5196, 43.8102) -> (-47.384, 43.8102) centre (-44.9518, 41.7693) ccw
  arc A172 (-77.0545, 8.3909) -> (-74.6223, 3.175) centre (-74.6223, 6.35) ccw
  arc A173 (-74.6223, 47.625) -> (-77.0545, 42.4091) centre (-74.6223, 44.45) ccw
  point P0 (-571.3006, 34.3975)
  point P1 (-581.025, 23.8125)
  point P2 (-581.025, 4.8134)
  point P3 (-581.025, 4.8134)
  point P4 (-565.0829, 26.9875)
  point P5 (-581.025, 26.9875)
  point P6 (-581.025, 45.9866)
  point P7 (-581.025, 45.9866)
  point P8 (-559.381, 20.1328)
  point P9 (-550.8435, 3.175)
  point P10 (-578.2551, 3.175)
  point P11 (-545.1517, 3.175)
  point P12 (-525.2277, 23.8125)
  point P13 (-12.8994, 34.3975)
  point P14 (-3.175, 23.8125)
  point P15 (-3.175, 4.8134)
  point P16 (-3.175, 4.8134)
  point P17 (-19.1171, 26.9875)
  point P18 (-3.175, 26.9875)
  point P19 (-3.175, 45.9866)
  point P20 (-3.175, 45.9866)
  point P21 (-24.819, 20.1328)
  point P22 (-25.2743, 19.5902)
  point P23 (-30.2527, 18.5966)
  point P24 (-5.9449, 3.175)
  point P25 (-30.2527, 32.2034)
  point P26 (-517.979, 20.1328)
  point P27 (-523.6809, 26.9875)
  point P28 (-509.4415, 3.175)
  point P29 (-483.8257, 23.8125)
  point P30 (-503.7497, 3.175)
  point P31 (-476.577, 20.1328)
  point P32 (-482.2789, 26.9875)
  point P33 (-468.0395, 3.175)
  point P34 (-442.4237, 23.8125)
  point P35 (-462.3477, 3.175)
  point P36 (-435.175, 20.1328)
  point P37 (-440.8769, 26.9875)
  point P38 (-426.6375, 3.175)
  point P39 (-401.0217, 23.8125)
  point P40 (-420.9457, 3.175)
  point P41 (-393.773, 20.1328)
  point P42 (-399.4749, 26.9875)
  point P43 (-385.2355, 3.175)
  point P44 (-359.6197, 23.8125)
  point P45 (-379.5437, 3.175)
  point P46 (-352.371, 20.1328)
  point P47 (-358.0729, 26.9875)
  point P48 (-343.8335, 3.175)
  point P49 (-318.2177, 23.8125)
  point P50 (-338.1417, 3.175)
  point P51 (-310.969, 20.1328)
  point P52 (-316.6709, 26.9875)
  point P53 (-302.4315, 3.175)
  point P54 (-276.8157, 23.8125)
  point P55 (-296.7397, 3.175)
  point P56 (-269.567, 20.1328)
  point P57 (-275.2689, 26.9875)
  point P58 (-261.0295, 3.175)
  point P59 (-235.4137, 23.8125)
  point P60 (-255.3377, 3.175)
  point P61 (-228.165, 20.1328)
  point P62 (-233.8669, 26.9875)
  point P63 (-219.6275, 3.175)
  point P64 (-194.0117, 23.8125)
  point P65 (-213.9357, 3.175)
  point P66 (-186.763, 20.1328)
  point P67 (-192.4649, 26.9875)
  point P68 (-178.2255, 3.175)
  point P69 (-152.6097, 23.8125)
  point P70 (-172.5337, 3.175)
  point P71 (-145.361, 20.1328)
  point P72 (-151.0629, 26.9875)
  point P73 (-136.8235, 3.175)
  point P74 (-111.2077, 23.8125)
  point P75 (-131.1317, 3.175)
  point P76 (-103.959, 20.1328)
  point P77 (-109.6609, 26.9875)
  point P78 (-95.4215, 3.175)
  point P79 (-69.8057, 23.8125)
  point P80 (-89.7297, 3.175)
  point P81 (-62.557, 20.1328)
  point P82 (-68.2589, 26.9875)
  point P83 (-54.0195, 3.175)
  point P84 (-28.4037, 23.8125)
  point P85 (-48.3277, 3.175)
  point P86 (-262.1465, 3.175)
  point P87 (-386.3525, 3.175)
  point P88 (-427.7545, 3.175)
  point P89 (-469.1565, 3.175)
  point P90 (-510.5585, 3.175)
  point P91 (-551.9605, 3.175)
  point P92 (-564.1356, 20.002)
  point P93 (-303.5485, 3.175)
  point P94 (-344.9505, 3.175)
  point P95 (-292.1, 26.9875)
  point P96 (-292.1, 44.682)
  point P97 (-220.7445, 3.175)
  point P98 (-179.3425, 3.175)
  point P99 (-159.4185, 23.8125)
  point P100 (-118.0165, 23.8125)
  point P101 (-137.9405, 3.175)
  point P102 (-96.5385, 3.175)
  point P103 (-55.1365, 3.175)
  point P104 (-20.0644, 20.002)
  point P105 (-32.2395, 3.175)
  point P106 (-20.7426, 3.175)
  dimension "d53" = 3.175
  dimension "d54" = 3.175
  dimension "d55" = 3.175
  dimension "d58" = 3.175
  dimension "d74" = 3.175
  dimension "d75" = 3.175
  dimension "d76" = 3.175
  dimension "d77" = 3.175
  dimension "d78" = 33.0962
  dimension "d79" = 50
  dimension "d80" = 3.175
  dimension "d83" = 41.402
  constraints: 702 end point, 348 point on circle, 174 centre point, 158 point on line, 79 symmetric about line, 29 tangent, 11 equal radius, 9 horizontal, 2 midpoint, 2 vertical, 1 collinear, 1 parallel, 1191 other
  measures "d53" distance between parallel lines of L4 L2
  measures "d54" radius of A0
  measures "d55" distance from line of point (-571.301, 34.398) L5
  measures "d58" radius of A3
  measures "d74" radius of A9
  measures "d75" distance between parallel lines of L23 L17
  measures "d76" distance between parallel lines of L24 L25
  measures "d77" diameter of L26 L1
  measures "d78" distance of L32.end point (-525.228, 23.812)
  measures "d79" angle of L29 L30
  measures "d80" radius of A12
  measures "d83" distance of L14.start L54.start
extrude "Extrusion5" cut sketch "Sketch5" against normal blind 46.0375 contours A95 L195 L193 A96 L194 L197 L13 | L13 L197 A94 L196 A95 | L13 L201 A98 L203 A99 | L2 A1 L3 A0 L5 A2 | A7 L7 A8 L8 A6 L6 | L9 A4 L11 A3 L10 A5 | A9 L19 L16 A11 L20 A10 L12 | A13 L26 L28 A14 L30 A12 L27 L25 | L33 A15 L35 A17 L34 A16 | A20 L38 A18 L37 A19 L36 | L39 A24 L41 A26 L40 A25 | A23 L44 A21 L43 A22 L42 | L45 A28 L49 A29 L46 L48 A27 | L56 A41 L57 A31 L55 A30 | L60 A32 L61 A40 L63 A33 | A36 L69 L72 A34 L71 A35 L70 L68 | L76 A38 L78 A39 L77 A37 | L81 A53 L82 A43 L80 A42 | L85 A44 L86 A52 L88 A45 | A48 L94 L97 A46 L96 A47 L95 L93 | L101 A50 L103 A51 L102 A49 | L106 A65 L107 A55 L105 A54 | L110 A56 L111 A64 L113 A57 | A60 L119 L122 A58 L121 A59 L120 L118 | L126 A62 L128 A63 L127 A61 | L131 A77 L132 A67 L130 A66 | L135 A68 L136 A76 L138 A69 | A72 L144 L147 A70 L146 A71 L145 L143 | L151 A74 L153 A75 L152 A73 | L156 A89 L157 A79 L155 A78 | L160 A80 L161 A88 L163 A81 | A84 L169 L172 A82 L171 A83 L170 L168 | L176 A86 L178 A87 L177 A85 | L181 A101 L182 A91 L180 A90 | L185 A92 L186 A100 L188 A93 | L206 A113 L207 A103 L205 A102 | L210 A104 L211 A112 L213 A105 | A108 L219 L222 A106 L221 A107 L220 L218 | L226 A110 L228 A111 L227 A109 | L231 A125 L232 A115 L230 A114 | L235 A116 L236 A124 L238 A117 | A120 L244 L247 A118 L246 A119 L245 L243 | L251 A122 L253 A123 L252 A121 | L256 A137 L257 A127 L255 A126 | L260 A128 L261 A136 L263 A129 | A132 L269 L272 A130 L271 A131 L270 L268 | L276 A134 L278 A135 L277 A133 | L281 A149 L282 A139 L280 A138 | L285 A140 L286 A148 L288 A141 | A144 L294 L297 A142 L296 A143 L295 L293 | L301 A146 L303 A147 L302 A145 | L306 A161 L307 A151 L305 A150 | L310 A152 L311 A160 L313 A153 | A156 L319 L322 A154 L321 A155 L320 L318 | L326 A158 L328 A159 L327 A157 | L331 A173 L332 A163 L330 A162 | L335 A164 L336 A172 L338 A165 | A168 L344 L347 A166 L346 A167 L345 L343 | L351 A170 L353 A171 L352 A169
equation "\"d3\" = Length"
equation "\"Length\" = 584.2"
body "Solid1"
